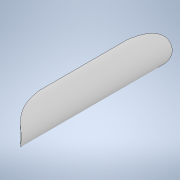
# Autodesk Inventor part: Segment_Deckel
Saved by Autodesk Inventor 2020 (Build 240168000, 168)
## iProperties
Created: 2022-01-25
Part Number: Segment_Deckel
Material: Generisch
Document SubType Name: Modeling
Designer: sp
Density: 1 g/cm^3
Appearance: Vorgabe
Author: sp
Autodesk Inventor part; units mm, degrees
ref_plane "YZ Plane" through (0, 0, 0) normal (1, 0, 0) x (0, 1, 0)
ref_plane "XZ Plane" through (0, 0, 0) normal (0, 1, 0) x (-1, 0, 0)
ref_plane "XY Plane" through (0, 0, 0) normal (0, 0, 1) x (1, 0, 0)
sketch "Skizze1" plane through (0, 0, 0) normal (0, 0, 1) x (1, 0, 0)
  circle A0 centre (0, 0) radius 33
  circle A1 centre (0, 0) radius 31
  dimension "d0" = 66
  dimension "d1" = 62
  constraints: 2 centre point, 2 coincident
  measures "d0" diameter of A0
  measures "d1" diameter of A1
extrude "Extrusion1" add sketch "Skizze1" along normal mid plane 300
sketch "Skizze2" plane through (0, 0, 0) normal (0, 1, 0) x (-1, 0, 0)
  line L0 (-10, 169.5773) -> (-10, -169.8146) construction
  line L1 (-74.8376, 0) -> (82.6362, 0) construction
  line L2 (-10, 75) -> (-10, -75)
  line L3 (-33, -150) -> (-33, 150) projected
  line L4 (33, 150) -> (-33, 150) projected
  line L5 (-33, -150) -> (33, -150) projected
  spline S0 degree 2 poles (-10, 75) (-18.0478, 153.5197) (-72.8449, 128.3193) knots 0 0 0 1 1 1
  spline S1 degree 2 poles (-10, -75) (-17.6631, -153.0376) (-74.8376, -130) knots 0 0 0 1 1 1
  line L6 (33, -150) -> (-33, -150)
  line L7 (33, -150) -> (33, 150)
  line L8 (33, -150) -> (33, 150) projected
  line L9 (33, 150) -> (-33, 150)
  line L10 (-33, 150) -> (-33, 130)
  line L11 (-33, -150) -> (-33, 150) projected
  line L12 (33, -150) -> (-33, -150)
  point P0 (0, 0)
  point P1 (-33, -130)
  dimension "d4" = 10
  dimension "d5" = 150
  dimension "d6" = 20
  dimension "d7" = 20
  constraints: 16 end point, 5 point on line, 4 collinear, 1 horizontal, 1 perpendicular, 1 symmetric about line, 1 vertical, 6 other
  measures "d4" distance from line of point (0, 0) L0
  measures "d5" distance of L2.start L2.end
  measures "d6" distance from line of L10.end L4
  measures "d7" distance from line of point (-33, -130) L5
extrude "Extrusion3" cut sketch "Skizze2" against normal mid plane 70 contours S0 L3 L4 L7 L5 S1 L2
